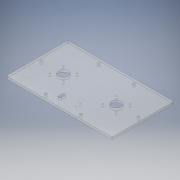
# Autodesk Inventor part: BT001_trajan20_21
Saved by Autodesk Inventor 2022.2 (Build 262287000, 287)
## iProperties
Company: HTBLA Kaindorf
RuleStatus: InUse
Created: 2022-08-03
Part Number: BT001_trajan20_21
Project: Zeichenmaschine_v2
Material: Acryl
Description: Platte Stepper Motoren
Document SubType Name: Modeling
Designer: trajan20
Density: 1.188 g/cm^3
Appearance: Transparent - farblos
Mass: 193.347 g
Surface Area: 707.029 cm^2
Volume: 162.75 cm^3
AfterDocNew0: iProperties-Editor_aufrufen
Author: jan
Keywords: 2021
Autodesk Inventor part; units mm, degrees
ref_plane "YZ Plane" through (0, 0, 0) normal (1, 0, 0) x (0, 1, 0)
ref_plane "XZ Plane" through (0, 0, 0) normal (0, 1, 0) x (-1, 0, 0)
ref_plane "XY Plane" through (0, 0, 0) normal (0, 0, 1) x (1, 0, 0)
sketch "Skizze3" plane through (0, 0, 0) normal (0, 0, 1) x (1, 0, 0)
  line L0 (0, 0) -> (-140, 0)
  line L1 (-140, 0) -> (-140, 120)
  line L2 (-140, 240) -> (0, 240)
  line L3 (0, 240) -> (0, 0)
  line L4 (-34.5565, 44.5) -> (-109.2584, 44.5) construction
  line L5 (-42.5521, 75.5) -> (-110.6291, 75.5) construction
  line L6 (-85.5, 104.3529) -> (-85.5, 36.2759) construction
  line L7 (-54.5, 102.2969) -> (-54.5, 32.1639) construction
  line L8 (-70, -15.9958) -> (-70, 12.0858) construction
  circle A0 centre (-70, 60) radius 11
  circle A1 centre (-85.5, 75.5) radius 1.5
  circle A2 centre (-85.5, 44.5) radius 1.5
  circle A3 centre (-54.5, 44.5) radius 1.5
  circle A4 centre (-54.5, 75.5) radius 1.5
  line L9 (-140, 120) -> (0, 120) construction
  line L10 (-140, 120) -> (-140, 240)
  line L11 (-139.4457, 80) -> (19.1397, 80) construction
  line L12 (12.4919, 138.4135) -> (-57.0145, 138.4135) construction
  line L13 (-20, 139.378) -> (-20, 104.3529) construction
  line L14 (-29.3, 147.764) -> (-29.3, 112.7389) construction
  line L15 (-20, 101.5865) -> (-29.3, 101.5865) construction
  line L16 (-20, 104.5865) -> (-29.3, 104.5865)
  line L17 (-29.3, 98.5865) -> (-20, 98.5865)
  arc A5 (-20, 98.5865) -> (-20, 104.5865) centre (-20, 101.5865) ccw
  arc A6 (-29.3, 104.5865) -> (-29.3, 98.5865) centre (-29.3, 101.5865) ccw
  line L18 (-6.3901, 160) -> (-134.3919, 160) construction
  point P0 (-70, 0)
  point P1 (-70, 10)
  point P2 (-130, 80)
  point P3 (-137.8382, 80)
  point P4 (-130, 160)
  point P5 (-10, 160)
  point P6 (-10, 80)
  point P7 (-70, 230)
  point P8 (-29.3, 138.4135)
  point P9 (-20, 138.4135)
  point P10 (-24.65, 101.5865)
  dimension "d4" = 240
  dimension "d5" = 140
  dimension "d6" = 31
  dimension "d7" = 31
  dimension "d8" = 15.5
  dimension "d9" = 15.5
  dimension "d10" = 60
  dimension "d11" = 22
  dimension "d12" = 3
  dimension "d13" = 3
  dimension "d14" = 3
  dimension "d15" = 3
  dimension "d22" = 10
  dimension "d23" = 10
  dimension "d24" = 10
  dimension "d25" = 10
  dimension "d26" = 10
  dimension "d34" = 10
  dimension "d35" = 9.3
  dimension "d36" = 18.4135
  dimension "d37" = 20
  dimension "d38" = 3
  dimension "d43" = 36.827
  dimension "d44" = 80
  dimension "d45" = 80
  constraints: 40 end point, 23 point on line, 7 centre point, 6 horizontal, 5 coincident, 5 parallel, 5 vertical, 4 point on circle, 4 tangent, 3 midpoint, 3 perpendicular
  measures "d4" distance between parallel lines of L2 L0
  measures "d5" distance between parallel lines of L1 L3
  measures "d6" distance between parallel lines of L6 L7
  measures "d7" distance between parallel lines of L5 L4
  measures "d8" distance from line of L7 point (-70, 60)
  measures "d9" distance from line of L5 point (-70, 60)
  measures "d10" distance from line of L0 point (-70, 60)
  measures "d11" diameter of A0
  measures "d12" diameter of A3
  measures "d13" diameter of A2
  measures "d14" diameter of A4
  measures "d15" diameter of A1
  measures "d22" distance from line of L0 point (-70, 10)
  measures "d23" distance from line of point (-10, 80) L3
  measures "d24" distance from line of L3 point (-10, 160)
  measures "d25" distance from line of L10 point (-130, 160)
  measures "d26" distance from line of L1 point (-130, 80)
  measures "d34" distance from line of L2 point (-70, 230)
  measures "d35" distance of point (-29.3, 138.414) point (-20, 138.414)
  measures "d36" distance between parallel lines of L9 L12
  measures "d37" distance between parallel lines of L13 L3
  measures "d38" radius of A6
  measures "d43" distance between parallel lines of L12 L15
  measures "d44" distance between parallel lines of L2 L18
  measures "d45" distance between parallel lines of L0 L11
extrude "Extrusion3" add sketch "Skizze3" against normal blind 5 contours L0 L1 L10 L2 L3 | A0 | A1 | A2 | A3 | A4 | A5 L17 A6 L16
fillet "Rundung1" radius 2 4 edges at (0, 0, -2.5) (0, 240, -2.5) (-140, 240, -2.5) (-140, 0, -2.5)
ref_plane "Arbeitsebene1" through (-140, 120, 0) normal (0, 1, 0) x (1, 0, 0)
extrude "Extrusion4" cut sketch "Skizze3" against normal through all contours A0 | A1 | A2 | A3 | A4
mirror "Spiegeln1" about plane through (-140, 120, 0) normal (0, 1, 0) of "Extrusion4"
hole "Bohrung1" at (-70, 60, 0) at (-70, 10, 0) at (-130, 80, 0) at (-130, 160, 0) at (-10, 160, 0) at (-10, 80, 0) at (-70, 230, 0) direction (0, 0, -1) diameter 5.5 end through all
extrude "Extrusion5" cut sketch "Skizze3" against normal blind 10 contours A5 L17 A6 L16
hole "Bohrung2" at (-20, 138.4135, 0) at (-29.3, 138.4135, 0) direction (0, 0, -1) diameter 1.567 depth 4 tip angle 118 thread size "M2x0.4" class "6H" standard "ISO Metric profile"
equation "\"d8\" = 0.5 * d6"
equation "\"d9\" = d8"
equation "\"d23\" = d22"
equation "\"d24\" = d23"
equation "\"d25\" = d22"
equation "\"d26\" = d25"
equation "\"d36\" = 0.5 * d43"
